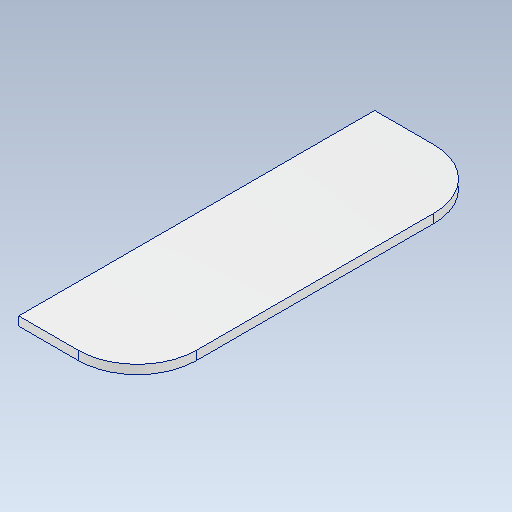
# Autodesk Inventor part: Shelf-ver1-1111-2021
Saved by Autodesk Inventor 2021 (Build 250183000, 183)
## iProperties
Created: 2021-03-03
Part Number: Shelf-ver1-1111-2021
Material: Aluminum 6061
Document SubType Name: Modeling
Designer: CMurray
Density: 2.7 g/cm^3
Appearance: Aluminum - Flat
Author: CMurray
Autodesk Inventor part; units mm, degrees
ref_plane "YZ Plane" through (0, 0, 0) normal (1, 0, 0) x (0, 1, 0)
ref_plane "XZ Plane" through (0, 0, 0) normal (0, 1, 0) x (-1, 0, 0)
ref_plane "XY Plane" through (0, 0, 0) normal (0, 0, 1) x (1, 0, 0)
sketch "Sketch1" plane through (0, 0, 0) normal (0, 1, 0) x (-1, 0, 0)
  line L0 (0, 0) -> (508, 0)
  line L1 (508, 0) -> (508, -1524)
  line L2 (508, -1524) -> (0, -1524)
  line L3 (0, -1524) -> (0, 0)
  dimension "d0" = 1524
  dimension "d1" = 508
  constraints: 8 end point, 2 parallel, 1 horizontal, 1 perpendicular
  measures "d0" distance between parallel lines of L2 L0
  measures "d1" distance between parallel lines of L3 L1
extrude "Extrusion1" add sketch "Sketch1" along normal blind 38.1
fillet "Fillet1" radius 254 1 edges at (0, 19.05, 0)
fillet "Fillet2" radius 254 1 edges at (0, 19.05, -1524)
sketch "Sketch2" plane through (0, 0, 0) normal (0, -1, 0) x (1, 0, 0)
  line L0 (-254, -1524) -> (-508, -1524) projected
  line L1 (-508, -1524) -> (-508, 0) projected
  line L2 (-508, -1524) -> (-508, 0)
  line L3 (-508, 0) -> (-508, -381)
  line L4 (-508, -381) -> (-444.5, -381)
  line L5 (-444.5, -381) -> (-444.5, -508)
  line L6 (-444.5, -508) -> (-508, -508)
  line L7 (-508, -1524) -> (-508, -1143)
  line L8 (-508, -1143) -> (-444.5, -1143)
  line L9 (-444.5, -1143) -> (-444.5, -1016)
  line L10 (-444.5, -1016) -> (-508, -1016)
  point P0 (0, 0)
  dimension "d6" = 381
  dimension "d7" = 63.5
  dimension "d8" = 127
  dimension "d9" = 381
  dimension "d10" = 127
  constraints: 18 end point, 5 perpendicular, 4 point on line, 2 vertical
  measures "d6" distance of L1.end L3.end
  measures "d7" distance of L3.end L4.end
  measures "d8" distance of L4.end L5.end
  measures "d9" distance of L0.end L7.end
  measures "d10" distance of L8.end L9.end
extrude "Extrusion2" add sketch "Sketch2" along normal blind 25.4
body "Solid1"
